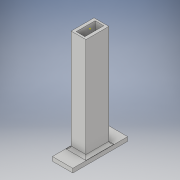
# Autodesk Inventor part: Bacon1
Saved by Autodesk Inventor 2018.2 (Build 222227000, 227)
## iProperties
Created: 2018-03-23
Part Number: Bacon1
Material: Generic
Document SubType Name: Modeling
Designer: MIABo
Density: 1 g/cm^3
Appearance: Default
Author: MIABo
Autodesk Inventor part; units mm, degrees
ref_plane "YZ Plane" through (0, 0, 0) normal (1, 0, 0) x (0, 1, 0)
ref_plane "XZ Plane" through (0, 0, 0) normal (0, 1, 0) x (-1, 0, 0)
ref_plane "XY Plane" through (0, 0, 0) normal (0, 0, 1) x (1, 0, 0)
sketch "Sketch1" plane through (0, 0, 0) normal (0, 1, 0) x (-1, 0, 0)
  line L0 (12.7, 34.1313) -> (-12.7, 34.1313)
  line L1 (-12.7, 34.1313) -> (-12.7, -34.1313)
  line L2 (-12.7, -34.1313) -> (12.7, -34.1313)
  line L3 (12.7, -34.1313) -> (12.7, 34.1313)
  line L4 (12.7, 34.1313) -> (-12.7, -34.1313) construction
  line L5 (-12.7, 34.1313) -> (12.7, -34.1313) construction
  point P0 (0, 0)
  dimension "d0" = 25.4
  dimension "d1" = 68.2625
  constraints: 12 end point, 2 midpoint, 2 parallel, 1 horizontal, 1 perpendicular
  measures "d0" distance of L2.end L1.end
  measures "d1" distance of L1.end L0.end
extrude "Extrusion1" add sketch "Sketch1" along normal blind 5.08
sketch "Sketch2" plane through (0, 5.08, 0) normal (0, 1, 0) x (1, 0, 0)
  line L0 (-5.3975, 11.7221) -> (5.3975, 11.7221)
  line L1 (5.3975, 11.7221) -> (5.3975, -11.7221)
  line L2 (5.3975, -11.7221) -> (-5.3975, -11.7221)
  line L3 (-5.3975, -11.7221) -> (-5.3975, 11.7221)
  line L4 (-5.3975, 11.7221) -> (5.3975, -11.7221) construction
  line L5 (5.3975, 11.7221) -> (-5.3975, -11.7221) construction
  line L6 (-9.2075, 14.2875) -> (9.2075, 14.2875)
  line L7 (9.2075, 14.2875) -> (9.2075, -14.2875)
  line L8 (9.2075, -14.2875) -> (-9.2075, -14.2875)
  line L9 (-9.2075, -14.2875) -> (-9.2075, 14.2875)
  line L10 (-9.2075, 14.2875) -> (9.2075, -14.2875) construction
  line L11 (9.2075, 14.2875) -> (-9.2075, -14.2875) construction
  point P0 (0, 0)
  dimension "d4" = 10.795
  dimension "d5" = 23.4442
  dimension "d6" = 18.415
  dimension "d7" = 28.575
  constraints: 24 end point, 4 midpoint, 4 parallel, 2 horizontal, 2 perpendicular
  measures "d4" distance of L1.end L2.end
  measures "d5" distance of L0.end L1.end
  measures "d6" distance of L7.end L8.end
  measures "d7" distance of L6.end L7.end
extrude "Extrusion2" add sketch "Sketch2" along normal blind 127
sketch "Sketch4" plane through (0, 132.08, 0) normal (0, 1, 0) x (1, 0, 0)
  point P0 (0, 0)
sketch "Sketch6" plane through (0, 5.08, 0) normal (0, 1, 0) x (1, 0, 0)
  point P0 (0, 0)
sketch "Sketch7" plane through (9.2075, 5.08, -14.2875) normal (0, 0, -1) x (-1, 0, 0)
  line L0 (-3.4925, 0) -> (21.9075, 0) projected
  circle A0 centre (9.2075, 12.7) radius 3.81
  point P0 (9.2075, -5.08)
  dimension "d13" = 12.7
  dimension "d14" = 7.62
  constraints: 1 centre point, 1 coincident
  measures "d13" distance from line of point (9.207, 12.7) L0
  measures "d14" diameter of A0
extrude "Extrusion4" cut sketch "Sketch7" against normal blind 5.08
fillet "Fillet1" radius 3.175 4 edges at (0, 5.08, -14.2875) (-9.2075, 5.08, 0) (0, 5.08, 14.2875) (9.2075, 5.08, 0)
body "Solid1"
